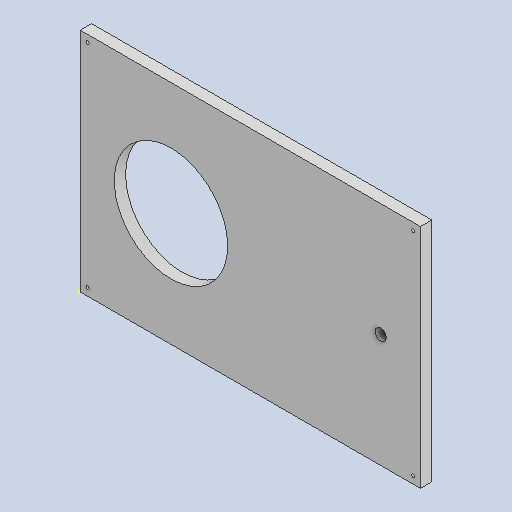
# Autodesk Inventor part: base cap
Saved by Autodesk Inventor 2022 (Build 260153000, 153)
## iProperties
Created: 2021-06-28
Part Number: base cap
Material: Generic
Document SubType Name: Sheet Metal
Designer: parag
Density: 1 g/cm^3
Sheet Metal Rule: Default_mm
Appearance: Default
Author: parag
Autodesk Inventor part; units mm, degrees
ref_plane "YZ Plane" through (0, 0, 0) normal (1, 0, 0) x (0, 1, 0)
ref_plane "XZ Plane" through (0, 0, 0) normal (0, 1, 0) x (-1, 0, 0)
ref_plane "XY Plane" through (0, 0, 0) normal (0, 0, 1) x (1, 0, 0)
sketch "Sketch1" plane through (0, 0, 0) normal (0, 0, 1) x (1, 0, 0)
  line L0 (0, 0) -> (300, 0)
  line L1 (300, 0) -> (300, 200)
  line L2 (300, 200) -> (0, 200)
  line L3 (0, 200) -> (0, 0)
  dimension "d0" = 300
  dimension "d1" = 200
  constraints: 8 end point, 2 parallel, 1 horizontal, 1 perpendicular
  measures "d0" distance between parallel lines of L1 L3
  measures "d1" distance between parallel lines of L0 L2
extrude "Extrusion1" add sketch "Sketch1" along normal blind 10
sketch "Sketch2" plane through (0, 0, 0) normal (0, 0, -1) x (-1, 0, 0)
  circle A0 centre (-80, 100) radius 50
  line L0 (-300, 200) -> (0, 200) projected
  line L1 (0, 200) -> (0, 0) projected
  dimension "d4" = 100
  dimension "d5" = 100
  dimension "d6" = 80
  constraints: 1 centre point
  measures "d4" diameter of A0
  measures "d5" distance from line of L0 A0.centre
  measures "d6" distance from line of L1 A0.centre
extrude "Extrusion2" cut sketch "Sketch2" against normal through all
sketch "Sketch3" plane through (0, 0, 10) normal (0, 0, 1) x (1, 0, 0)
  point P0 (0, 0)
sketch "Sketch4" plane through (0, 0, 10) normal (0, 0, 1) x (1, 0, 0)
  circle A0 centre (265, 100) radius 5
  line L0 (0, 0) -> (300, 0) projected
  line L1 (300, 0) -> (300, 200) projected
  dimension "d9" = 10
  dimension "d10" = 100
  dimension "d11" = 30
  constraints: 1 centre point
  measures "d9" diameter of A0
  measures "d10" distance from line of A0.centre L0
  measures "d11" distance edge to line of A0 L1
extrude "Extrusion3" cut sketch "Sketch4" against normal through all
sketch "Sketch5" plane through (0, 0, 0) normal (0, 0, -1) x (-1, 0, 0)
  circle A0 centre (-6.4515, 6.4515) radius 1.4515
  circle A1 centre (-293.5485, 193.5485) radius 1.4515
  circle A2 centre (-293.5485, 6.4515) radius 1.4515
  line L0 (0, 200) -> (0, 0) projected
  line L1 (0, 0) -> (-300, 0) projected
  circle A3 centre (-6.4515, 193.5485) radius 1.4515
  line L2 (-300, 200) -> (0, 200) projected
  line L3 (-300, 0) -> (-300, 200) projected
  dimension "d14" = 2.903
  dimension "d16" = 2.903
  dimension "d17" = 2.903
  dimension "d18" = 5
  dimension "d19" = 5
  dimension "d20" = 2.903
  dimension "d21" = 5
  dimension "d22" = 5
  dimension "d23" = 5
  dimension "d24" = 5
  dimension "d25" = 5
  dimension "d26" = 5
  constraints: 4 centre point
  measures "d14" diameter of A0
  measures "d16" diameter of A1
  measures "d17" diameter of A2
  measures "d18" distance edge to line of A0 L0
  measures "d19" distance edge to line of A0 L1
  measures "d20" diameter of A3
  measures "d21" distance edge to line of A3 L0
  measures "d22" distance edge to line of A3 L2
  measures "d23" distance edge to line of A1 L3
  measures "d24" distance edge to line of A1 L2
  measures "d25" distance edge to line of A2 L3
  measures "d26" distance edge to line of A2 L1
extrude "Extrusion4" cut sketch "Sketch5" against normal through all contours A0 | A1 | A2 | A3
equation "\"BendRadius\" = Thickness"
equation "\"BendReliefWidth\" = Thickness"
equation "\"BendReliefDepth\" = 0.5 * Thickness"
equation "\"CornerReliefSize\" = 4 * Thickness"
equation "\"MinimumRemnant\" = 2 * Thickness"
equation "\"TransitionRadius\" = BendRadius"
equation "\"JacobiRadiusSize\" = BendRadius"
equation "\"GapSize\" = Thickness"
equation "\"Thickness\" = 0.5"
body "Solid1"
